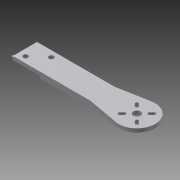
# Autodesk Inventor part: Arm2
Saved by Autodesk Inventor 2015 (Build 190159000, 159)
## iProperties
Created: 2016-01-15
Part Number: Arm2
Material: ABS Plastic
Document SubType Name: Modeling
Designer: 576994
Density: 1.06 g/cm^3
Appearance: Smooth - White
Mass: 8.89196 g
Surface Area: 57.7874 cm^2
Volume: 8.38864 cm^3
Author: 576994
Autodesk Inventor part; units mm, degrees
ref_plane "YZ Plane" through (0, 0, 0) normal (1, 0, 0) x (0, 1, 0)
ref_plane "XZ Plane" through (0, 0, 0) normal (0, 1, 0) x (-1, 0, 0)
ref_plane "XY Plane" through (0, 0, 0) normal (0, 0, 1) x (1, 0, 0)
sketch "Sketch1" plane through (0, 0, 0) normal (0, 0, 1) x (1, 0, 0)
  line L0 (0, 0) -> (64, 0)
  line L1 (64, 20) -> (0, 20)
  line L2 (0, 20) -> (0, 0)
  arc A0 (89.7812, -4.7516) -> (89.7812, 24.7516) centre (92.5, 10) ccw
  line L3 (64, 20) -> (89.7812, 24.7516)
  line L4 (64, 0) -> (89.7812, -4.7516)
  circle A1 centre (92.5, 10) radius 1.5
  dimension "d5" = 30
  dimension "d6" = 92.5
  dimension "d9" = 3
  dimension "d26" = 20
  constraints: 10 end point, 2 centre point, 2 coincident, 2 point on circle, 2 tangent, 1 horizontal, 1 parallel
  measures "d5" diameter of A0
  measures "d6" distance from line of L2 A0.centre
  measures "d9" diameter of A1
  measures "d26" distance of L1.end L0.start
extrude "Extrusion1" add sketch "Sketch1" along normal blind 3 contours L2 L1 L3 A0 L4 L0 | A1
extrude "Extrusion2" cut sketch "Sketch1" along normal blind 10 contours A1
sketch "Sketch3" plane through (0, 0, 3) normal (0, 0, 1) x (1, 0, 0)
  circle A0 centre (92.5, 10) radius 1.5 projected
  circle A1 centre (92.5, 10) radius 1.5
  line L0 (92.5, 10) -> (128.0101, 10) construction
  arc A2 (96.8308, 16.1692) -> (98.6692, 14.3308) centre (97.75, 15.25) ccw
  arc A3 (100.5192, 16.1808) -> (98.6808, 18.0192) centre (99.6, 17.1) ccw
  line L1 (96.8308, 16.1692) -> (98.6808, 18.0192)
  line L2 (100.5192, 16.1808) -> (98.6692, 14.3308)
  point P0 (0, 0)
  dimension "d18" = 2.6
  dimension "d19" = 2.6
  constraints: 6 end point, 4 point on circle, 3 centre point, 1 coincident, 1 horizontal, 1 parallel
  measures "d18" diameter of A2
  measures "d19" diameter of A3
extrude "Extrusion3" cut sketch "Sketch3" against normal blind 10 contours L1 A3 L2 A2
pattern_circular "Circular Pattern1" count 4 over 360 about axis through (92.5, 10, 0) along (0, 0, 1) of "Extrusion3"
sketch "Sketch4" plane through (0, 0, 3) normal (0, 0, 1) x (1, 0, 0)
  circle A0 centre (5.625, 5) radius 1.6
  circle A1 centre (16.875, 15) radius 1.6
  point P0 (0, 0)
  dimension "d27" = 3.2
  dimension "d28" = 3.2
  constraints: 2 centre point
  measures "d27" diameter of A0
  measures "d28" diameter of A1
extrude "Extrusion4" cut sketch "Sketch4" against normal blind 10
sketch "Sketch5" plane through (0, 0, 3) normal (0, 0, 1) x (1, 0, 0)
  line L0 (91.1147, 10.2457) -> (94, 10)
  circle A0 centre (92.5, 10) radius 1.5 projected
  circle A1 centre (16.875, 15) radius 1.6 projected
  line L1 (17.5362, 16.511) -> (16.875, 15)
  circle A2 centre (5.625, 5) radius 1.6 projected
  line L2 (16.875, 15) -> (5.625, 5)
  circle A3 centre (16.875, 15) radius 2.032
  circle A4 centre (5.625, 5) radius 2.032
  point P0 (0, 0)
  dimension "d31" = 4.064
  dimension "d32" = 4.064
  constraints: 6 end point, 2 centre point, 2 coincident, 1 horizontal alignment, 1 other
  measures "d31" diameter of A3
  measures "d32" diameter of A4
extrude "Extrusion5" cut sketch "Sketch5" against normal blind 10 contours A1 L2 L1 | A3 | A2 | A4 | L1 L2 A1
sketch "Sketch6" plane through (0, 0, 3) normal (0, 0, 1) x (1, 0, 0)
  circle A0 centre (92.5, 10) radius 1.5 projected
  line L0 (92.8215, 11.4329) -> (92.5, 10)
  circle A1 centre (92.5, 10) radius 3.0734
  point P0 (0, 0)
  dimension "d35" = 6.1468
  constraints: 2 end point, 1 centre point, 1 coincident
  measures "d35" diameter of A1
extrude "Extrusion6" cut sketch "Sketch6" against normal blind 10
sketch "Sketch7" plane through (0, 0, 3) normal (0, 0, 1) x (1, 0, 0)
  point P0 (0, 0)
sketch "Sketch8" plane through (0, 0, 3) normal (0, 0, 1) x (1, 0, 0)
  point P0 (0, 0)
sketch "Sketch9" plane through (0, 0, 3) normal (0, 0, 1) x (1, 0, 0)
  point P0 (0, 0)
sketch "Sketch11" plane through (0, 0, 0) normal (0, 0, -1) x (-1, 0, 0)
  line L0 (0, 0) -> (-64, 0) projected
  line L1 (-22.5, 0) -> (-22.5, 20)
  line L2 (-64, 20) -> (0, 20) projected
  line L3 (0, 20) -> (0, 0) projected
  line L4 (-64, 0) -> (-64, 20)
  dimension "d42" = 22.5
  constraints: 4 end point, 2 point on line, 2 vertical
  measures "d42" distance between parallel lines of L3 L1
extrude "Extrusion8" add sketch "Sketch11" along normal blind 2 contours L0 L4 L2 L1
fillet "Fillet2" radius 2 1 edges at (64, 10, -2)
body "Solid1"
